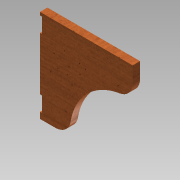
# Autodesk Inventor part: Z Holdere
Saved by Autodesk Inventor 2014 (Build 180170000, 170)
## iProperties
Created: 2015-05-11
Part Number: Z Holdere
Material: Wood (Cherry)
Document SubType Name: Modeling
Designer: Mathias Lyngklip Kjeldgaard
Density: 0.63 g/cm^3
Appearance: Cherry - Natural Low Gloss
Mass: 104.101 g
Surface Area: 341.923 cm^2
Volume: 165.239 cm^3
Author: Mathias Lyngklip Kjeldgaard
Autodesk Inventor part; units mm, degrees
ref_plane "YZ Plane" through (0, 0, 0) normal (1, 0, 0) x (0, 1, 0)
ref_plane "XZ Plane" through (0, 0, 0) normal (0, 1, 0) x (-1, 0, 0)
ref_plane "XY Plane" through (0, 0, 0) normal (0, 0, 1) x (1, 0, 0)
sketch "Sketch1" plane through (0, 0, 0) normal (0, 1, 0) x (-1, 0, 0)
  line L0 (0, -12) -> (150, -12)
  line L1 (150, -12) -> (-170, -12)
  line L2 (150, -12) -> (150, 0)
  line L3 (-170, 0) -> (150, 0)
  line L4 (-170, -12) -> (-170, 0)
  arc A0 (0, -37) -> (21.03, -61.6828) centre (25, -37) ccw
  line L5 (0, -12) -> (0, -37)
  arc A1 (100.3172, -140.97) -> (125, -162) centre (125, -137) ccw
  line L6 (150, -162) -> (125, -162)
  arc A2 (100.3172, -140.97) -> (21.03, -61.6828) centre (5.8332, -156.1668) ccw
  line L7 (150, -17) -> (146.5, -17)
  line L8 (146.5, -17) -> (146.5, -41.5)
  line L9 (146.5, -41.5) -> (150, -41.5)
  line L10 (150, -127.5) -> (146.5, -127.5)
  line L11 (146.5, -127.5) -> (146.5, -152)
  line L12 (146.5, -152) -> (150, -152)
  line L13 (150, -12) -> (150, -17)
  line L14 (150, -41.5) -> (150, -127.5)
  line L15 (150, -152) -> (150, -162)
  line L16 (162.5, -20.3274) -> (147.5, -20.3274)
  line L17 (147.5, -37.698) -> (162.5, -37.698)
  line L18 (147.5, -40.746) -> (162.5, -40.746)
  line L19 (162.246, -41) -> (147.754, -41)
  line L20 (147.754, -17) -> (162.246, -17)
  line L21 (162.5, -17.254) -> (147.5, -17.254)
  line L22 (147.5, -20.3274) -> (147.5, -37.698) construction
  point P0 (0, 0)
extrude "Tykkelse af plade" add sketch "Sketch1" along normal blind 12 contours L0 L13 L7 L8 L9 L14 L10 L11 L12 L15 L6 A1 A2 A0 L5
equation "\"d12\" = d9"
equation "\"d13\" = d16"
equation "\"d9\" = 24.5"
equation "\"d16\" = 3.5"
body "Solid1"
